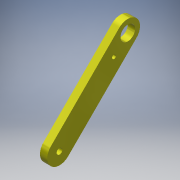
# Autodesk Inventor part: torque arm
Saved by Autodesk Inventor 2017 (Build 210142000, 142)
## iProperties
Created: 2017-01-17
Part Number: torque arm
Material: Generic
Document SubType Name: Modeling
Designer: Ben
Density: 1 g/cm^3
Appearance: Smooth - Yellow
Author: Ben
Autodesk Inventor part; units mm, degrees
ref_plane "YZ Plane" through (0, 0, 0) normal (1, 0, 0) x (0, 1, 0)
ref_plane "XZ Plane" through (0, 0, 0) normal (0, 1, 0) x (-1, 0, 0)
ref_plane "XY Plane" through (0, 0, 0) normal (0, 0, 1) x (1, 0, 0)
sketch "Sketch1" plane through (0, 0, 0) normal (1, 0, 0) x (0, 1, 0)
  circle A0 centre (0, 0) radius 6.35
  circle A1 centre (-44.45, 44.45) radius 1.905
  arc A2 (-40.1924, 49.1612) -> (-49.1612, 40.1924) centre (-44.45, 44.45) ccw
  arc A3 (-7.0668, -6.3864) -> (6.3864, 7.0668) centre (0, 0) ccw
  line L0 (0, 0) -> (0, -9.525) construction
  line L1 (0, 0) -> (-44.45, 44.45) construction
  line L2 (0, 0) -> (-44.45, -44.45) construction
  line L3 (0, 0) -> (-64.9365, 0) construction
  line L4 (-44.45, 44.45) -> (-48.9401, 48.9401) construction
  circle A4 centre (-8.9803, 8.9803) radius 1.27
  line L5 (-49.1612, 40.1924) -> (-7.0668, -6.3864)
  line L6 (6.3864, 7.0668) -> (-40.1924, 49.1612)
  dimension "d0" = 12.7
  dimension "d1" = 3.81
  dimension "d10" = 12.7
  dimension "d15" = 88.9
  dimension "d16" = 2.54
  dimension "d17" = 12.7
  dimension "d18" = 9.525
  constraints: 14 end point, 6 point on circle, 5 centre point, 4 tangent, 3 coincident, 2 perpendicular, 1 horizontal, 1 point on line, 1 vertical, 1 other
  measures "d0" diameter of A0
  measures "d1" diameter of A1
  measures "d10" diameter of A2
  measures "d15" distance of L2.end A1.centre
  measures "d16" diameter of A4
  measures "d17" distance of point (0, 0) A4.centre
  measures "d18" radius of A3
extrude "Extrusion1" add sketch "Sketch1" along normal blind 4.7625
body "Solid1"
